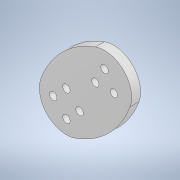
# Autodesk Inventor part: 駆動節
Saved by Autodesk Inventor 2022.2 (Build 262287000, 287)
## iProperties
Created: 2022-01-08
Part Number: 駆動節
Material: Aluminum 2014-T6
Document SubType Name: Modeling
Designer: acps
Density: 2.78927 g/cm^3
Appearance: Satin
Author: acps
Autodesk Inventor part; units mm, degrees
ref_plane "YZ Plane" through (0, 0, 0) normal (1, 0, 0) x (0, 1, 0)
ref_plane "XZ Plane" through (0, 0, 0) normal (0, 1, 0) x (-1, 0, 0)
ref_plane "XY Plane" through (0, 0, 0) normal (0, 0, 1) x (1, 0, 0)
sketch "Sketch2" plane through (0, 0, 0) normal (0, 0, 1) x (1, 0, 0)
  line L0 (-12.7279, -12.7279) -> (0, 0) construction
  line L1 (-12.7279, -12.7279) -> (-7.4558, -12.7279) construction
  line L2 (-12.7279, -12.7279) -> (0, 0) construction
  line L3 (-17.252, -29.9799) -> (-9.2664, -21.9943) construction
  line L4 (-2.9446, 9.7833) -> (-10.9302, 1.7977) construction
  arc A0 (-21.1882, -9.6582) -> (-9.6582, -21.1882) centre (-12.7279, -12.7279) ccw
  arc A1 (8.4603, -3.0697) -> (-3.0697, 8.4603) centre (0, 0) ccw
  circle A2 centre (-8.3439, -12.7279) radius 1.25
  circle A3 centre (-8.3439, -12.7279) radius 3.1 construction
  circle A4 centre (-12.7279, -8.3439) radius 1.25
  circle A5 centre (-12.7279, -8.3439) radius 3.1 construction
  circle A6 centre (-17.112, -12.7279) radius 1.25
  circle A7 centre (-17.112, -12.7279) radius 3.1 construction
  circle A8 centre (-12.7279, -17.112) radius 1.25
  circle A9 centre (-12.7279, -17.112) radius 3.1 construction
  circle A10 centre (-3.1, -1.7898) radius 1.25
  circle A11 centre (-3.1, -1.7898) radius 3.1 construction
  circle A12 centre (3.1, -1.7898) radius 3.1 construction
  circle A13 centre (3.1, -1.7898) radius 1.25
  circle A14 centre (0, 3.5796) radius 3.1 construction
  circle A15 centre (0, 3.5796) radius 1.25
  arc A16 (-9.6582, -21.1882) -> (8.4603, -3.0697) centre (-19.9758, 7.2478) ccw
  line L5 (1.4142, -14.1421) -> (-6.364, -6.364) construction
  arc A17 (-3.0697, 8.4603) -> (-21.1882, -9.6582) centre (7.2478, -19.9758) ccw
  point P0 (-6.364, -6.364)
  dimension "d34" = 18
  dimension "d35" = 9
  dimension "d36" = 2.5
  dimension "d37" = 6.2
  dimension "d38" = 360
  dimension "d39" = 2.5
  dimension "d40" = 6.2
  dimension "d41" = 360
  dimension "d42" = 11
  dimension "d43" = 45
  constraints: 18 centre point, 14 end point, 9 point on circle, 8 coincident, 8 tangent, 3 symmetric about line, 2 midpoint, 1 horizontal, 1 horizontal alignment, 1 parallel, 1 perpendicular, 1 vertical alignment, 31 other
  measures "d34" distance of L0.start L0.end
  measures "d35" radius of A1
  measures "d36" diameter of A2
  measures "d37" diameter of A3
  measures "d39" diameter of A10
  measures "d40" diameter of A11
  measures "d42" distance of L5.start L5.end
  measures "d43" angle of L1 L0
extrude "Extrusion2" add sketch "Sketch2" along normal blind 3
body "Solid2"
